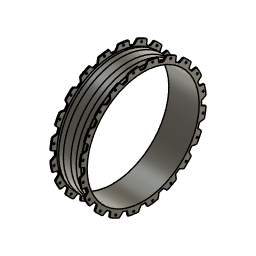
primary_turbine_case_eng_model (Autodesk Fusion 360 design; units mm, degrees)
Autodesk Fusion 360 part; units mm, degrees
sketch "Sketch1" plane through (0, 0, 0) normal (0, 1, 0) x (1, 0, 0)
  line L0 (0, 0) -> (130, 0) construction
  line L1 (130, 0) -> (130, -240) construction
  line L2 (130, -240) -> (0, -240) construction
  line L3 (0, -240) -> (0, 0) construction
  line L4 (110, 0) -> (110, -328.3547) construction
  line L5 (0, -240) -> (130, -240) construction
  line L6 (130, -240) -> (0, -240)
  line L7 (130, -240) -> (130, -249.1409)
  line L8 (130, -249.1409) -> (130, -270)
  line L9 (130, -270) -> (125, -270)
  line L10 (125, -270) -> (125, -245)
  line L11 (0, -240) -> (0, -245.4084)
  line L12 (0, -245.4084) -> (0, -270)
  line L13 (0, -270) -> (5, -270)
  line L14 (5, -270) -> (5, -245)
  line L15 (15, -245) -> (15, -247)
  line L16 (15, -247) -> (35, -247)
  line L17 (35, -247) -> (65, -245)
  line L18 (90, -245) -> (90, -247)
  line L19 (90, -247) -> (110, -247)
  line L20 (110, -245) -> (110, -247)
  line L21 (110, -245) -> (125, -245)
  line L22 (5, -245) -> (15, -245)
  line L23 (65, -245) -> (90, -245)
  dimension "d1" = 130
  dimension "d2" = 240
  dimension "d3" = 20
  dimension "d4" = 5
  dimension "d5" = 5
  dimension "d6" = 5
  dimension "d7" = 270
  dimension "d8" = 270
  dimension "d9" = 10
  dimension "d10" = 2
  dimension "d11" = 20
  dimension "d12" = 30
  dimension "d13" = 25
  dimension "d14" = 20
  dimension "d15" = 7
  constraint horizontal L0
  constraint vertical L1
  constraint horizontal L2
  constraint vertical L3
  constraint coincident L0.start L3.end
  constraint coincident L0 L4.start
  constraint perpendicular L2 L4
  constraint perpendicular L5 L8
  constraint perpendicular L8 L9
  constraint perpendicular L5 L10
  constraint perpendicular L2 L12
  constraint perpendicular L12 L13
  constraint perpendicular L2 L14
  constraint perpendicular L14 L22
  constraint perpendicular L15 L22
  constraint perpendicular L15 L16
  constraint perpendicular L18 L22
  constraint perpendicular L4 L19
  constraint coincident L20.start L22
  constraint coincident L4 L20.start
  constraint perpendicular L19 L20
  constraint collinear L21 L22
  constraint coincident L17.end L22
  constraint collinear L22 L23
  measures "d1" distance of L0.start L0.end
  measures "d2" distance of L2 L0.start
  measures "d3" distance of L1 L4
  measures "d4" distance of L12.end L13.end
  measures "d5" distance of L8.end L9.end
  measures "d6" distance of L2 L22
  measures "d7" distance of L0.start L13
  measures "d8" distance of L0 L9
  measures "d9" distance of L14 L15
  measures "d10" distance of L16 L22
  measures "d11" distance of L15.end L16.end
  measures "d12" horizontal distance of L16.end L17.end
  measures "d13" distance of L17.end L18
  measures "d14" distance of L18.end L19.end
  measures "d15" distance of L6 L19
revolve "Revolve1" add sketch "Sketch1" angle 360 about axis through (0, 0, 0) along (1, 0, 0)
sketch "Sketch2" plane through (0, 0, 0) normal (1, 0, 0) x (0, 1, 0)
  circle A0 centre (0, 0) radius 270
  circle A1 centre (0, 0) radius 250
  line L0 (0, 0) -> (0, 356.9599) construction
  line L1 (0, 275.8256) -> (0, 242.615) construction
  line L2 (-10, 275.8256) -> (-10, 242.615) construction
  line L3 (10, 275.8256) -> (10, 242.615) construction
  line L4 (-20, 275.8256) -> (-20, 242.615) construction
  line L5 (20, 275.8256) -> (20, 242.615) construction
  line L6 (20, 269.2582) -> (10, 249.7999)
  line L7 (-10, 249.7999) -> (-20, 269.2582)
  point P0 (20, 269.2582)
  point P1 (10, 249.7999)
  point P2 (-10, 249.7999)
  point P3 (-20, 269.2582)
  dimension "d17" = 500
  dimension "d18" = 10
  dimension "d19" = -10
  dimension "d20" = 20
  dimension "d21" = -20
  constraint concentric A0 A1
  constraint coincident A0.centre A1.centre
  constraint vertical L0
  constraint coincident L0 L1.start
  constraint coincident L0 L1.end
  constraint coincident L5 P0
  constraint coincident A0 P0
  constraint coincident L3 P1
  constraint coincident A1 P1
  constraint coincident A1 P2
  constraint coincident L2 P2
  constraint coincident A0 P3
  constraint coincident L4 P3
  constraint coincident P0 L6.start
  constraint coincident P1 L6.end
  constraint coincident P2 L7.start
  constraint coincident P3 L7.end
  measures "d17" diameter of A1
extrude "Extrude1" cut sketch "Sketch2" along normal blind 160 contours A0 A1 L6 L7 picked at (12.224, 262.9919)
pattern_circular "C-Pattern1" count 20 over 360 about axis through (1.75, 0, 0) along (1, 0, 0) of "Extrude1"
sketch "Sketch3" plane through (0, 0, 0) normal (-1, 0, 0) x (0, -1, 0)
  line L0 (-64.1842, 262.2601) -> (-67.6819, 240.664)
  arc A0 (-67.6819, 240.664) -> (-86.703, 234.4837) centre (0, 0) ccw
  line L1 (-86.703, 234.4837) -> (-102.2265, 249.8995)
  arc A1 (-102.2265, 249.8995) -> (-142.0857, 229.5902) centre (0, 0) ccw
  line L2 (-142.0857, 229.5902) -> (-138.7385, 207.9702)
  arc A2 (-138.7385, 207.9702) -> (-154.9189, 196.2145) centre (0, 0) ccw
  line L3 (-154.9189, 196.2145) -> (-174.4464, 206.0788)
  arc A3 (-174.4464, 206.0788) -> (-206.0788, 174.4464) centre (0, 0) ccw
  line L4 (-206.0788, 174.4464) -> (-196.2145, 154.9189)
  arc A4 (-196.2145, 154.9189) -> (-207.9702, 138.7385) centre (0, 0) ccw
  line L5 (-207.9702, 138.7385) -> (-229.5902, 142.0857)
  arc A5 (-229.5902, 142.0857) -> (-249.8995, 102.2265) centre (0, 0) ccw
  line L6 (-249.8995, 102.2265) -> (-234.4837, 86.703)
  arc A6 (-234.4837, 86.703) -> (-240.664, 67.6819) centre (0, 0) ccw
  line L7 (-240.664, 67.6819) -> (-262.2601, 64.1842)
  arc A7 (-262.2601, 64.1842) -> (-269.2582, 20) centre (0, 0) ccw
  line L8 (-269.2582, 20) -> (-249.7999, 10)
  arc A8 (-249.7999, 10) -> (-249.7999, -10) centre (0, 0) ccw
  line L9 (-249.7999, -10) -> (-269.2582, -20)
  arc A9 (-269.2582, -20) -> (-262.2601, -64.1842) centre (0, 0) ccw
  line L10 (-262.2601, -64.1842) -> (-240.664, -67.6819)
  arc A10 (-240.664, -67.6819) -> (-234.4837, -86.703) centre (0, 0) ccw
  line L11 (-234.4837, -86.703) -> (-249.8995, -102.2265)
  arc A11 (-249.8995, -102.2265) -> (-229.5902, -142.0857) centre (0, 0) ccw
  line L12 (-229.5902, -142.0857) -> (-207.9702, -138.7385)
  arc A12 (-207.9702, -138.7385) -> (-196.2145, -154.9189) centre (0, 0) ccw
  line L13 (-196.2145, -154.9189) -> (-206.0788, -174.4464)
  arc A13 (-206.0788, -174.4464) -> (-174.4464, -206.0788) centre (0, 0) ccw
  line L14 (-174.4464, -206.0788) -> (-154.9189, -196.2145)
  arc A14 (-154.9189, -196.2145) -> (-138.7385, -207.9702) centre (0, 0) ccw
  line L15 (-138.7385, -207.9702) -> (-142.0857, -229.5902)
  arc A15 (-142.0857, -229.5902) -> (-102.2265, -249.8995) centre (0, 0) ccw
  line L16 (-102.2265, -249.8995) -> (-86.703, -234.4837)
  arc A16 (-86.703, -234.4837) -> (-67.6819, -240.664) centre (0, 0) ccw
  line L17 (-67.6819, -240.664) -> (-64.1842, -262.2601)
  arc A17 (-64.1842, -262.2601) -> (-20, -269.2582) centre (0, 0) ccw
  line L18 (-20, -269.2582) -> (-10, -249.7999)
  arc A18 (-10, -249.7999) -> (10, -249.7999) centre (0, 0) ccw
  line L19 (10, -249.7999) -> (20, -269.2582)
  arc A19 (20, -269.2582) -> (64.1842, -262.2601) centre (0, 0) ccw
  line L20 (64.1842, -262.2601) -> (67.6819, -240.664)
  arc A20 (67.6819, -240.664) -> (86.703, -234.4837) centre (0, 0) ccw
  line L21 (86.703, -234.4837) -> (102.2265, -249.8995)
  arc A21 (102.2265, -249.8995) -> (142.0857, -229.5902) centre (0, 0) ccw
  line L22 (142.0857, -229.5902) -> (138.7385, -207.9702)
  arc A22 (138.7385, -207.9702) -> (154.9189, -196.2145) centre (0, 0) ccw
  line L23 (154.9189, -196.2145) -> (174.4464, -206.0788)
  arc A23 (174.4464, -206.0788) -> (206.0788, -174.4464) centre (0, 0) ccw
  line L24 (206.0788, -174.4464) -> (196.2145, -154.9189)
  arc A24 (196.2145, -154.9189) -> (207.9702, -138.7385) centre (0, 0) ccw
  line L25 (207.9702, -138.7385) -> (229.5902, -142.0857)
  arc A25 (229.5902, -142.0857) -> (249.8995, -102.2265) centre (0, 0) ccw
  line L26 (249.8995, -102.2265) -> (234.4837, -86.703)
  arc A26 (234.4837, -86.703) -> (240.664, -67.6819) centre (0, 0) ccw
  line L27 (240.664, -67.6819) -> (262.2601, -64.1842)
  arc A27 (262.2601, -64.1842) -> (269.2582, -20) centre (0, 0) ccw
  line L28 (269.2582, -20) -> (249.7999, -10)
  arc A28 (249.7999, -10) -> (249.7999, 10) centre (0, 0) ccw
  line L29 (249.7999, 10) -> (269.2582, 20)
  arc A29 (269.2582, 20) -> (262.2601, 64.1842) centre (0, 0) ccw
  line L30 (262.2601, 64.1842) -> (240.664, 67.6819)
  arc A30 (240.664, 67.6819) -> (234.4837, 86.703) centre (0, 0) ccw
  line L31 (234.4837, 86.703) -> (249.8995, 102.2265)
  arc A31 (249.8995, 102.2265) -> (229.5902, 142.0857) centre (0, 0) ccw
  line L32 (229.5902, 142.0857) -> (207.9702, 138.7385)
  arc A32 (207.9702, 138.7385) -> (196.2145, 154.9189) centre (0, 0) ccw
  line L33 (196.2145, 154.9189) -> (206.0788, 174.4464)
  arc A33 (206.0788, 174.4464) -> (174.4464, 206.0788) centre (0, 0) ccw
  line L34 (174.4464, 206.0788) -> (154.9189, 196.2145)
  arc A34 (154.9189, 196.2145) -> (138.7385, 207.9702) centre (0, 0) ccw
  line L35 (138.7385, 207.9702) -> (142.0857, 229.5902)
  arc A35 (142.0857, 229.5902) -> (102.2265, 249.8995) centre (0, 0) ccw
  line L36 (102.2265, 249.8995) -> (86.703, 234.4837)
  arc A36 (86.703, 234.4837) -> (67.6819, 240.664) centre (0, 0) ccw
  line L37 (67.6819, 240.664) -> (64.1842, 262.2601)
  arc A37 (64.1842, 262.2601) -> (20, 269.2582) centre (0, 0) ccw
  line L38 (20, 269.2582) -> (10, 249.7999)
  arc A38 (10, 249.7999) -> (-10, 249.7999) centre (0, 0) ccw
  line L39 (-10, 249.7999) -> (-20, 269.2582)
  arc A39 (-20, 269.2582) -> (-64.1842, 262.2601) centre (0, 0) ccw
  circle A40 centre (0, 0) radius 240
  line L40 (0, 0) -> (48.2446, 304.6041) construction
  circle A41 centre (0, 0) radius 260 construction
  circle A42 centre (40.673, 256.799) radius 4
  dimension "d26" = 29.2005
  dimension "d27" = 58.4009
  dimension "d28" = 520
  dimension "d29" = 8
  constraint coincident A0.centre A1.centre
  constraint coincident L40 A42.centre
  constraint coincident A41 A42.centre
  measures "d26" distance of L38.end L40
  measures "d27" distance of A36.end L38.end
  measures "d28" diameter of A41
  measures "d29" diameter of A42
extrude "Extrude2" cut sketch "Sketch3" against normal blind 220 contours A42
pattern_circular "C-Pattern2" count 20 over 360 about axis through (1.75, 0, 0) along (1, 0, 0) of "Extrude2"
sketch "Sketch4" plane through (0, 0, 0) normal (0, 1, 0) x (1, 0, 0)
  point P0 (110, 0)
  point P1 (110, 0)
  constraint coincident P0 P1
sketch "Sketch5" plane through (130, 0, 0) normal (1, 0, 0) x (0, 1, 0)
  circle A0 centre (40.6729, 256.799) radius 4
  circle A1 centre (118.0375, 231.6617) radius 4
  circle A2 centre (183.8477, 183.8478) radius 4
  circle A3 centre (231.6617, 118.0376) radius 4
  circle A4 centre (256.799, 40.673) radius 4
  circle A5 centre (256.799, -40.6729) radius 4
  circle A6 centre (231.6617, -118.0375) radius 4
  circle A7 centre (183.8478, -183.8477) radius 4
  circle A8 centre (118.0376, -231.6617) radius 4
  circle A9 centre (40.673, -256.799) radius 4
  circle A10 centre (-40.6729, -256.799) radius 4
  circle A11 centre (-118.0375, -231.6617) radius 4
  circle A12 centre (-183.8477, -183.8478) radius 4
  circle A13 centre (-231.6617, -118.0376) radius 4
  circle A14 centre (-256.799, -40.673) radius 4
  circle A15 centre (-256.799, 40.6729) radius 4
  circle A16 centre (-231.6617, 118.0375) radius 4
  circle A17 centre (-183.8478, 183.8477) radius 4
  circle A18 centre (-118.0376, 231.6617) radius 4
  circle A19 centre (-40.673, 256.799) radius 4
  line L0 (67.6819, 240.664) -> (64.1842, 262.2601)
  arc A20 (64.1842, 262.2601) -> (20, 269.2582) centre (0, 0) ccw
  line L1 (20, 269.2582) -> (10, 249.7999)
  arc A21 (10, 249.7999) -> (-10, 249.7999) centre (0, 0) ccw
  line L2 (-10, 249.7999) -> (-20, 269.2582)
  arc A22 (-20, 269.2582) -> (-64.1842, 262.2601) centre (0, 0) ccw
  line L3 (-64.1842, 262.2601) -> (-67.6819, 240.664)
  arc A23 (-67.6819, 240.664) -> (-86.703, 234.4837) centre (0, 0) ccw
  line L4 (-86.703, 234.4837) -> (-102.2265, 249.8995)
  arc A24 (-102.2265, 249.8995) -> (-142.0857, 229.5902) centre (0, 0) ccw
  line L5 (-142.0857, 229.5902) -> (-138.7385, 207.9702)
  arc A25 (-138.7385, 207.9702) -> (-154.9189, 196.2145) centre (0, 0) ccw
  line L6 (-154.9189, 196.2145) -> (-174.4464, 206.0788)
  arc A26 (-174.4464, 206.0788) -> (-206.0788, 174.4464) centre (0, 0) ccw
  line L7 (-206.0788, 174.4464) -> (-196.2145, 154.9189)
  arc A27 (-196.2145, 154.9189) -> (-207.9702, 138.7385) centre (0, 0) ccw
  line L8 (-207.9702, 138.7385) -> (-229.5902, 142.0857)
  arc A28 (-229.5902, 142.0857) -> (-249.8995, 102.2265) centre (0, 0) ccw
  line L9 (-249.8995, 102.2265) -> (-234.4837, 86.703)
  arc A29 (-234.4837, 86.703) -> (-240.664, 67.6819) centre (0, 0) ccw
  line L10 (-240.664, 67.6819) -> (-262.2601, 64.1842)
  arc A30 (-262.2601, 64.1842) -> (-269.2582, 20) centre (0, 0) ccw
  line L11 (-269.2582, 20) -> (-249.7999, 10)
  arc A31 (-249.7999, 10) -> (-249.7999, -10) centre (0, 0) ccw
  line L12 (-249.7999, -10) -> (-269.2582, -20)
  arc A32 (-269.2582, -20) -> (-262.2601, -64.1842) centre (0, 0) ccw
  line L13 (-262.2601, -64.1842) -> (-240.664, -67.6819)
  arc A33 (-240.664, -67.6819) -> (-234.4837, -86.703) centre (0, 0) ccw
  line L14 (-234.4837, -86.703) -> (-249.8995, -102.2265)
  arc A34 (-249.8995, -102.2265) -> (-229.5902, -142.0857) centre (0, 0) ccw
  line L15 (-229.5902, -142.0857) -> (-207.9702, -138.7385)
  arc A35 (-207.9702, -138.7385) -> (-196.2145, -154.9189) centre (0, 0) ccw
  line L16 (-196.2145, -154.9189) -> (-206.0788, -174.4464)
  arc A36 (-206.0788, -174.4464) -> (-174.4464, -206.0788) centre (0, 0) ccw
  line L17 (-174.4464, -206.0788) -> (-154.9189, -196.2145)
  arc A37 (-154.9189, -196.2145) -> (-138.7385, -207.9702) centre (0, 0) ccw
  line L18 (-138.7385, -207.9702) -> (-142.0857, -229.5902)
  arc A38 (-142.0857, -229.5902) -> (-102.2265, -249.8995) centre (0, 0) ccw
  line L19 (-102.2265, -249.8995) -> (-86.703, -234.4837)
  arc A39 (-86.703, -234.4837) -> (-67.6819, -240.664) centre (0, 0) ccw
  line L20 (-67.6819, -240.664) -> (-64.1842, -262.2601)
  arc A40 (-64.1842, -262.2601) -> (-20, -269.2582) centre (0, 0) ccw
  line L21 (-20, -269.2582) -> (-10, -249.7999)
  arc A41 (-10, -249.7999) -> (10, -249.7999) centre (0, 0) ccw
  line L22 (10, -249.7999) -> (20, -269.2582)
  arc A42 (20, -269.2582) -> (64.1842, -262.2601) centre (0, 0) ccw
  line L23 (64.1842, -262.2601) -> (67.6819, -240.664)
  arc A43 (67.6819, -240.664) -> (86.703, -234.4837) centre (0, 0) ccw
  line L24 (86.703, -234.4837) -> (102.2265, -249.8995)
  arc A44 (102.2265, -249.8995) -> (142.0857, -229.5902) centre (0, 0) ccw
  line L25 (142.0857, -229.5902) -> (138.7385, -207.9702)
  arc A45 (138.7385, -207.9702) -> (154.9189, -196.2145) centre (0, 0) ccw
  line L26 (154.9189, -196.2145) -> (174.4464, -206.0788)
  arc A46 (174.4464, -206.0788) -> (206.0788, -174.4464) centre (0, 0) ccw
  line L27 (206.0788, -174.4464) -> (196.2145, -154.9189)
  arc A47 (196.2145, -154.9189) -> (207.9702, -138.7385) centre (0, 0) ccw
  line L28 (207.9702, -138.7385) -> (229.5902, -142.0857)
  arc A48 (229.5902, -142.0857) -> (249.8995, -102.2265) centre (0, 0) ccw
  line L29 (249.8995, -102.2265) -> (234.4837, -86.703)
  arc A49 (234.4837, -86.703) -> (240.664, -67.6819) centre (0, 0) ccw
  line L30 (240.664, -67.6819) -> (262.2601, -64.1842)
  arc A50 (262.2601, -64.1842) -> (269.2582, -20) centre (0, 0) ccw
  line L31 (269.2582, -20) -> (249.7999, -10)
  arc A51 (249.7999, -10) -> (249.7999, 10) centre (0, 0) ccw
  line L32 (249.7999, 10) -> (269.2582, 20)
  arc A52 (269.2582, 20) -> (262.2601, 64.1842) centre (0, 0) ccw
  line L33 (262.2601, 64.1842) -> (240.664, 67.6819)
  arc A53 (240.664, 67.6819) -> (234.4837, 86.703) centre (0, 0) ccw
  line L34 (234.4837, 86.703) -> (249.8995, 102.2265)
  arc A54 (249.8995, 102.2265) -> (229.5902, 142.0857) centre (0, 0) ccw
  line L35 (229.5902, 142.0857) -> (207.9702, 138.7385)
  arc A55 (207.9702, 138.7385) -> (196.2145, 154.9189) centre (0, 0) ccw
  line L36 (196.2145, 154.9189) -> (206.0788, 174.4464)
  arc A56 (206.0788, 174.4464) -> (174.4464, 206.0788) centre (0, 0) ccw
  line L37 (174.4464, 206.0788) -> (154.9189, 196.2145)
  arc A57 (154.9189, 196.2145) -> (138.7385, 207.9702) centre (0, 0) ccw
  line L38 (138.7385, 207.9702) -> (142.0857, 229.5902)
  arc A58 (142.0857, 229.5902) -> (102.2265, 249.8995) centre (0, 0) ccw
  line L39 (102.2265, 249.8995) -> (86.703, 234.4837)
  arc A59 (86.703, 234.4837) -> (67.6819, 240.664) centre (0, 0) ccw
  circle A60 centre (0, 0) radius 240
  constraint coincident A20.centre A21.centre
equation "d7 = ( 540 / 2 ) * 1 mm"
equation "d8 = ( 540 / 2 ) * 1 mm"
equation "d26 = ( 58.401 / 2 ) * 1 mm"
